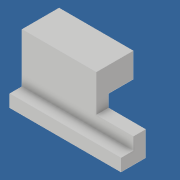
# Autodesk Inventor part: Part4
Saved by Autodesk Inventor 2018 (Build 220112000, 112)
## iProperties
Created: 2017-12-05
Part Number: Part4
Material: Generic
Document SubType Name: Modeling
Designer: 232963
Density: 1 g/cm^3
Appearance: Default
Author: 232963
Autodesk Inventor part; units mm, degrees
ref_plane "YZ Plane" through (0, 0, 0) normal (1, 0, 0) x (0, 1, 0)
ref_plane "XZ Plane" through (0, 0, 0) normal (0, 1, 0) x (-1, 0, 0)
ref_plane "XY Plane" through (0, 0, 0) normal (0, 0, 1) x (1, 0, 0)
sketch "Sketch1" plane through (0, 0, 0) normal (0, 0, 1) x (1, 0, 0)
  line L0 (-61.3765, 63.5) -> (14.8235, 63.5)
  line L1 (52.9235, 25.4) -> (52.9235, 0)
  line L2 (52.9235, 0) -> (-61.3765, 0)
  line L3 (-61.3765, 0) -> (-61.3765, 63.5)
  line L4 (52.9235, 25.4) -> (14.8235, 25.4)
  line L5 (14.8235, 25.4) -> (14.8235, 63.5)
  point P0 (0, 0)
  dimension "d0" = 38.1
  dimension "d1" = 76.2
  dimension "d2" = 38.1
  dimension "d3" = 114.3
  dimension "d4" = 63.5
  dimension "d5" = 25.4
  constraints: 12 end point, 2 parallel, 1 horizontal, 1 perpendicular
  measures "d0" distance of L4.end L0.end
  measures "d1" distance of L0.start L0.end
  measures "d2" distance of L1.start L4.end
  measures "d3" distance of L1.end L2.end
  measures "d4" distance of L2.end L0.start
  measures "d5" distance of L1.start L1.end
extrude "Extrusion1" add sketch "Sketch1" along normal blind 12.7
sketch "Sketch2" plane through (0, 0, 12.7) normal (0, 0, 1) x (1, 0, 0)
  line L0 (-61.3765, 0) -> (52.9235, 0) projected
  line L1 (-61.3765, 63.5) -> (-61.3765, 0) projected
  line L2 (52.9235, 0) -> (-61.3765, 0)
  line L3 (-61.3765, 0) -> (-61.3765, 12.7)
  line L4 (-61.3765, 12.7) -> (52.9235, 12.7)
  line L5 (52.9235, 12.7) -> (52.9235, 0)
  point P0 (0, 0)
  dimension "d8" = 12.7
  constraints: 8 end point, 2 parallel, 1 horizontal, 1 perpendicular, 1 point on line
  measures "d8" distance between parallel lines of L0 L4
extrude "Extrusion2" add sketch "Sketch2" along normal blind 12.7
sketch "Sketch3" plane through (0, 0, 0) normal (0, 0, -1) x (-1, 0, 0)
  line L0 (61.3765, 63.5) -> (61.3765, 12.7) projected
  line L1 (-14.8235, 25.4) -> (-14.8235, 63.5) projected
  line L2 (61.3765, 63.5) -> (-14.8235, 63.5)
  line L3 (-14.8235, 63.5) -> (-14.8235, 38.1)
  line L4 (-14.8235, 38.1) -> (61.3765, 38.1)
  line L5 (61.3765, 38.1) -> (61.3765, 63.5)
  point P0 (0, 0)
  dimension "d11" = 25.4
  constraints: 8 end point, 2 parallel, 1 horizontal, 1 perpendicular, 1 point on line
  measures "d11" distance between parallel lines of L2 L4
extrude "Extrusion3" add sketch "Sketch3" along normal blind 25.4
body "Solid1"
